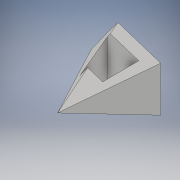
# Autodesk Inventor part: Деталь_3-19
Saved by Autodesk Inventor 2019.3 (Build 233278000, 278)
## iProperties
Created: 2020-03-15
Part Number: Деталь_3-19
Material: Типовые
Document SubType Name: Modeling
Designer: Diana
Density: 1 g/cm^3
Appearance: По умолчанию
Author: Diana
Autodesk Inventor part; units mm, degrees
ref_plane "YZ Plane" through (0, 0, 0) normal (1, 0, 0) x (0, 1, 0)
sketch "Эскиз1" plane through (0, 0, 0) normal (0, 0, 1) x (1, 0, 0)
  line L0 (-42.5, 0) -> (-13.1332, 40.4199)
  line L1 (-13.1332, 40.4199) -> (34.3832, 24.9809)
  line L2 (34.3832, 24.9809) -> (34.3832, -24.9809)
  line L3 (34.3832, -24.9809) -> (-13.1332, -40.4199)
  line L4 (-13.1332, -40.4199) -> (-42.5, 0)
  point P0 (0, 0)
  point P1 (0, 0)
  constraints: 10 end point, 1 coincident, 1 horizontal alignment, 12 other
ref_plane "РабПлоскость1" through (0, 0, 80) normal (0, 0, 1) x (1, 0, 0)
sketch "Эскиз2" plane through (0, 0, 80) normal (0, 0, 1) x (1, 0, 0)
  point P0 (0, 0)
  point P1 (0, 0)
  constraints: 1 coincident
loft "Лофт1" add profiles "Эскиз1" section 2 point at (0, 0, 80)
ref_plane "РабПлоскость2" through (0, -74.25, 0) normal (0, 1, 0) x (-1, 0, 0)
sketch "Эскиз3" plane through (0, -74.25, 0) normal (0, 1, 0) x (-1, 0, 0)
  line L0 (15, 40) -> (-10, 40)
  line L1 (-10, 10) -> (15, 10)
  line L2 (15, 10) -> (15, 40)
  line L3 (-10, 40) -> (-20, 10)
  line L4 (-20, 10) -> (-10, 10)
  point P0 (0, 0)
  point P1 (0, 80)
  point P2 (42.5, 0)
  point P3 (13.1332, 0)
  point P4 (-34.3832, 0)
  dimension "d7" = 25
  dimension "d8" = 30
  dimension "d9" = 15
  dimension "d10" = 35
  dimension "d11" = 10
  constraints: 10 end point, 2 horizontal, 1 parallel
  measures "d7" distance of L0.end L0.start
  measures "d8" distance of L1.end L0.start
  measures "d9" horizontal distance of L1.end point (0, 0)
  measures "d10" distance of L3.end L1.end
  measures "d11" vertical distance of point (0, 0) L1.end
extrude "Выдавливание1" cut sketch "Эскиз3" along normal through all
